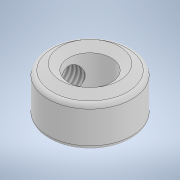
# Autodesk Inventor part: 5mm Collar
Saved by Autodesk Inventor 2022 (Build 260153000, 153)
## iProperties
Created: 2022-03-21
Part Number: 5mm Collar
Material: Generic
Document SubType Name: Modeling
Designer: Nick
Density: 1 g/cm^3
Appearance: Default
Author: Nick
Autodesk Inventor part; units mm, degrees
ref_plane "YZ Plane" through (0, 0, 0) normal (1, 0, 0) x (0, 1, 0)
ref_plane "XZ Plane" through (0, 0, 0) normal (0, 1, 0) x (-1, 0, 0)
ref_plane "XY Plane" through (0, 0, 0) normal (0, 0, 1) x (1, 0, 0)
sketch "Sketch1" plane through (0, 0, 0) normal (0, 0, 1) x (1, 0, 0)
  line L0 (2.55, 4.8) -> (3.525, 5.5)
  line L1 (3.525, 5.5) -> (4.5, 4.8)
  line L2 (4.5, 4.8) -> (5, 4.8)
  line L3 (5, 4.8) -> (5, 0)
  line L4 (5, 0) -> (2.55, 0)
  line L5 (2.55, 0) -> (2.55, 4.8)
  line L6 (0, 0) -> (0, 15.358) construction
  line L7 (2.55, 4.8) -> (4.5, 4.8) construction
  point P0 (3.775, 0)
  dimension "d0" = 2.55
  dimension "d1" = 5
  dimension "d2" = 5.5
  dimension "d4" = 4.8
  dimension "d5" = 0.5
  constraints: 16 end point, 3 perpendicular, 1 equal length, 1 horizontal, 1 horizontal alignment, 1 midpoint, 1 vertical
  measures "d0" distance between parallel lines of L5 L6
  measures "d1" distance between parallel lines of L6 L3
  measures "d2" distance from line of L4 L0.end
  measures "d4" distance between parallel lines of L4 L2
  measures "d5" distance of L1.end L2.end
revolve "Revolution1" add sketch "Sketch1" angle 360 about axis through (0, 0, 0) along (0, 1, 0)
fillet "Fillet1" radius 0.5 2 edges at (-5, 4.8, 0) (-5, 0, 0)
sketch "Sketch2" plane through (0, 0, 0) normal (1, 0, 0) x (0, 1, 0)
  circle A0 centre (2.4833, 0) radius 1.5
  point P0 (0, 0)
  dimension "d8" = 3
  constraints: 1 centre point
  measures "d8" diameter of A0
extrude "Extrusion1" cut sketch "Sketch2" against normal blind 10
thread "Thread1" size "M3x0.5" class "6H" standard "ANSI Metric M Profile" full length
body "Solid1"
